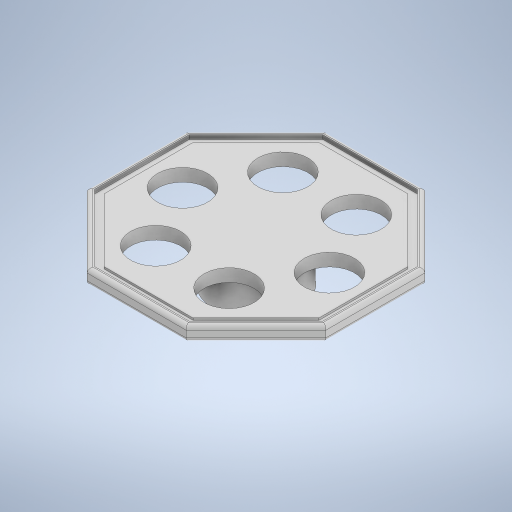
# Autodesk Inventor part: OV-PAM_top_2
Saved by Autodesk Inventor 2024 (Build 280153000, 153)
## iProperties
Created: 2023-06-16
Part Number: OV-PAM_top_2
Material: 일반
Document SubType Name: Modeling
Designer: jsw
Density: 1 g/cm^3
Appearance: 기본값
Author: jsw
Autodesk Inventor part; units mm, degrees
ref_plane "YZ Plane" through (0, 0, 0) normal (1, 0, 0) x (0, 1, 0)
ref_plane "XZ Plane" through (0, 0, 0) normal (0, 1, 0) x (-1, 0, 0)
ref_plane "XY Plane" through (0, 0, 0) normal (0, 0, 1) x (1, 0, 0)
sketch "스케치3" plane through (0, 0, 0) normal (0, 1, 0) x (-1, 0, 0)
  line L0 (35.7919, -14.8255) -> (14.8255, -35.7919)
  line L1 (14.8255, -35.7919) -> (-14.8255, -35.7919)
  line L2 (-14.8255, -35.7919) -> (-35.7919, -14.8255)
  line L3 (-35.7919, -14.8255) -> (-35.7919, 14.8255)
  line L4 (-35.7919, 14.8255) -> (-14.8255, 35.7919)
  line L5 (-14.8255, 35.7919) -> (14.8255, 35.7919)
  line L6 (14.8255, 35.7919) -> (35.7919, 14.8255)
  line L7 (35.7919, 14.8255) -> (35.7919, -14.8255)
  line L8 (32.5919, -13.5) -> (13.5, -32.5919)
  line L9 (13.5, -32.5919) -> (-13.5, -32.5919)
  line L10 (-13.5, -32.5919) -> (-32.5919, -13.5)
  line L11 (-32.5919, -13.5) -> (-32.5919, 13.5)
  line L12 (-32.5919, 13.5) -> (-13.5, 32.5919)
  line L13 (-13.5, 32.5919) -> (13.5, 32.5919)
  line L14 (13.5, 32.5919) -> (32.5919, 13.5)
  line L15 (32.5919, 13.5) -> (32.5919, -13.5)
  point P0 (0, 0)
  point P1 (0, 0)
  point P2 (0, 0)
  point P3 (0, 0)
  dimension "d43" = 27
  dimension "d44" = 3.2
  constraints: 32 end point, 3 coincident, 2 horizontal, 34 other
  measures "d43" distance of L8.end L9.end
  measures "d44" distance between parallel lines of L7 L15
extrude "돌출2" add sketch "스케치3" along normal blind 4.4 contours L0 L1 L2 L3 L4 L5 L6 L7 | L8 L9 L10 L11 L12 L13 L14 L15
sketch "스케치4" plane through (0, 4.4, 0) normal (0, 1, 0) x (1, 0, 0)
  line L0 (13.5, -32.5919) -> (-13.5, -32.5919)
  line L1 (-13.5, -32.5919) -> (-32.5919, -13.5)
  line L2 (-32.5919, -13.5) -> (-32.5919, 13.5)
  line L3 (-32.5919, 13.5) -> (-13.5, 32.5919)
  line L4 (-13.5, 32.5919) -> (13.5, 32.5919)
  line L5 (13.5, 32.5919) -> (32.5919, 13.5)
  line L6 (32.5919, 13.5) -> (32.5919, -13.5)
  line L7 (32.5919, -13.5) -> (13.5, -32.5919)
  line L8 (-14.1627, 34.1919) -> (14.1627, 34.1919)
  line L9 (14.1627, 34.1919) -> (34.1919, 14.1627)
  line L10 (34.1919, 14.1627) -> (34.1919, -14.1627)
  line L11 (34.1919, -14.1627) -> (14.1627, -34.1919)
  line L12 (14.1627, -34.1919) -> (-14.1627, -34.1919)
  line L13 (-14.1627, -34.1919) -> (-34.1919, -14.1627)
  line L14 (-34.1919, -14.1627) -> (-34.1919, 14.1627)
  line L15 (-34.1919, 14.1627) -> (-14.1627, 34.1919)
  line L16 (-13.3343, 32.1919) -> (13.3343, 32.1919)
  line L17 (13.3343, 32.1919) -> (32.1919, 13.3343)
  line L18 (32.1919, 13.3343) -> (32.1919, -13.3343)
  line L19 (32.1919, -13.3343) -> (13.3343, -32.1919)
  line L20 (13.3343, -32.1919) -> (-13.3343, -32.1919)
  line L21 (-13.3343, -32.1919) -> (-32.1919, -13.3343)
  line L22 (-32.1919, -13.3343) -> (-32.1919, 13.3343)
  line L23 (-32.1919, 13.3343) -> (-13.3343, 32.1919)
  line L24 (-35.7919, 14.8255) -> (-35.7919, -14.8255) projected
  point P0 (0, 0)
  point P1 (0, 0)
  point P2 (0, 0)
  point P3 (0, 0)
  dimension "d7" = 27
  dimension "d60" = 1.6
  dimension "d61" = 2
  constraints: 48 end point, 3 coincident, 3 horizontal, 51 other
  measures "d7" distance of L1.end L2.end
  measures "d60" distance between parallel lines of L14 L24
  measures "d61" distance between parallel lines of L14 L22
extrude "돌출3" cut sketch "스케치4" against normal blind 1.2 contours L0 L1 L2 L3 L4 L5 L6 L7 | L8 L9 L10 L11 L12 L13 L14 L15 | L16 L17 L18 L19 L20 L21 L22 L23
sketch "스케치9" plane through (0, 3.2, 0) normal (0, 1, 0) x (1, 0, 0)
  line L0 (-13.3343, 32.1919) -> (13.3343, 32.1919)
  line L1 (13.3343, 32.1919) -> (32.1919, 13.3343)
  line L2 (32.1919, 13.3343) -> (32.1919, -13.3343)
  line L3 (32.1919, -13.3343) -> (13.3343, -32.1919)
  line L4 (13.3343, -32.1919) -> (-13.3343, -32.1919)
  line L5 (-13.3343, -32.1919) -> (-32.1919, -13.3343)
  line L6 (-32.1919, -13.3343) -> (-32.1919, 13.3343)
  line L7 (-32.1919, 13.3343) -> (-13.3343, 32.1919)
  line L8 (-14.1627, 34.1919) -> (14.1627, 34.1919) projected
  line L9 (-12.0917, 29.1919) -> (12.0917, 29.1919)
  line L10 (12.0917, 29.1919) -> (29.1919, 12.0917)
  line L11 (29.1919, 12.0917) -> (29.1919, -12.0917)
  line L12 (29.1919, -12.0917) -> (12.0917, -29.1919)
  line L13 (12.0917, -29.1919) -> (-12.0917, -29.1919)
  line L14 (-12.0917, -29.1919) -> (-29.1919, -12.0917)
  line L15 (-29.1919, -12.0917) -> (-29.1919, 12.0917)
  line L16 (-29.1919, 12.0917) -> (-12.0917, 29.1919)
  point P0 (0, 0)
  point P1 (0, 0)
  point P2 (0, 0)
  dimension "d46" = 2
  dimension "d47" = 3
  constraints: 32 end point, 2 coincident, 2 horizontal, 34 other
  measures "d46" distance between parallel lines of L0 L8
  measures "d47" distance between parallel lines of L0 L9
extrude "돌출8" add sketch "스케치9" along normal blind 0.6 contours L0 L1 L2 L3 L4 L5 L6 L7 | L9 L10 L11 L12 L13 L14 L15 L16
fillet "모깎기1" radius 1.2 16 edges at (-35.7919, 4.4, 0) (-25.3087, 4.4, 25.3087) (0, 4.4, 35.7919) (25.3087, 4.4, 25.3087) (35.7919, 4.4, 0) (25.3087, 4.4, -25.3087) (0, 4.4, -35.7919) (-25.3087, 4.4, -25.3087) (25.3087, 0, 25.3087) (0, 0, 35.7919) (-25.3087, 0, 25.3087) (-35.7919, 0, 0) (-25.3087, 0, -25.3087) (0, 0, -35.7919) (25.3087, 0, -25.3087) (35.7919, 0, 0)
sketch "스케치11" plane through (0, 0, 0) normal (0, -1, 0) x (1, 0, 0)
  circle A0 centre (0, 0) radius 12.7
  dimension "d62" = 25.4
  constraints: 1 centre point, 1 coincident
  measures "d62" diameter of A0
extrude "돌출11" add sketch "스케치11" along normal blind 10.16
sketch "스케치12" plane through (0, -10.16, 0) normal (0, -1, 0) x (1, 0, 0)
  circle A0 centre (0, 0) radius 4.5
  line L0 (4.5, 2.5981) -> (4.5, -2.5981)
  line L1 (4.5, -2.5981) -> (0, -5.1962)
  line L2 (0, -5.1962) -> (-4.5, -2.5981)
  line L3 (-4.5, -2.5981) -> (-4.5, 2.5981)
  line L4 (-4.5, 2.5981) -> (0, 5.1962)
  line L5 (0, 5.1962) -> (4.5, 2.5981)
  point P0 (2.25, 3.8971)
  point P1 (-2.25, 3.8971)
  point P2 (4.5, 0)
  point P3 (-4.5, 0)
  point P4 (-2.25, -3.8971)
  point P5 (2.25, -3.8971)
  dimension "d65" = 9
  constraints: 12 end point, 2 coincident, 1 centre point, 1 tangent, 1 vertical, 13 other
  measures "d65" diameter of A0
extrude "돌출12" cut sketch "스케치12" against normal blind 12
sketch "스케치13" plane through (0, 0, 0) normal (0, -1, 0) x (1, 0, 0)
  circle A0 centre (-22, 0) radius 7.5
  circle A1 centre (-11, -19.0526) radius 7.5
  circle A2 centre (11, -19.0526) radius 7.5
  circle A3 centre (22, 0) radius 7.5
  circle A4 centre (11, 19.0526) radius 7.5
  circle A5 centre (-11, 19.0526) radius 7.5
  point P0 (0, 0)
  dimension "d70" = 15
  dimension "d71" = 22
  dimension "d74" = 360
  constraints: 6 centre point, 1 horizontal alignment, 13 other
  measures "d70" diameter of A0
  measures "d71" distance of A0.centre point (0, 0)
extrude "돌출13" cut sketch "스케치13" against normal up to surface (3.8 mm away)
sketch "스케치18" plane through (0, 1.84, 0) normal (0, -1, 0) x (1, 0, 0)
  line L0 (4.5, 2.5981) -> (4.5, -2.5981) projected
  line L1 (0, 5.1962) -> (4.5, 2.5981) projected
  line L2 (-4.5, 2.5981) -> (0, 5.1962) projected
  line L3 (-4.5, -2.5981) -> (-4.5, 2.5981) projected
  line L4 (0, -5.1962) -> (-4.5, -2.5981) projected
  line L5 (4.5, -2.5981) -> (0, -5.1962) projected
  line L6 (3.5, 2.0207) -> (3.5, -2.0207)
  line L7 (3.5, -2.0207) -> (0, -4.0415)
  line L8 (0, -4.0415) -> (-3.5, -2.0207)
  line L9 (-3.5, -2.0207) -> (-3.5, 2.0207)
  line L10 (-3.5, 2.0207) -> (0, 4.0415)
  line L11 (0, 4.0415) -> (3.5, 2.0207)
  point P0 (0, 0)
  point P1 (0, 0)
  dimension "d116" = 1
  constraints: 12 end point, 1 coincident, 1 vertical, 13 other
  measures "d116" distance between parallel lines of L6 L0
extrude "돌출14" add sketch "스케치18" along normal blind 8.5
fillet "모깎기2" radius 0.5 6 edges at (2.25, -10.16, 3.8971) (-2.25, -10.16, 3.8971) (4.5, -10.16, 0) (2.25, -10.16, -3.8971) (-2.25, -10.16, -3.8971) (-4.5, -10.16, 0)
equation "\"d85\" = 55deg"
equation "\"d105\" = 55deg"
